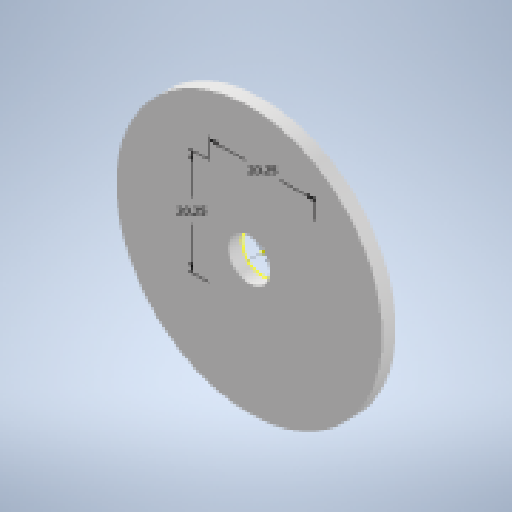
# Autodesk Inventor part: Base
Saved by Autodesk Inventor 2026 (Build 300175050, 175E)
## iProperties
Created: 2025-10-07
Part Number: Base
Material: Generic
Document SubType Name: Modeling
Designer: Cupri
Density: 1 g/cm^3
Appearance: Default
Author: Cupri
Autodesk Inventor part; units mm, degrees
ref_plane "YZ Plane" through (0, 0, 0) normal (1, 0, 0) x (0, 1, 0)
ref_plane "XZ Plane" through (0, 0, 0) normal (0, 1, 0) x (-1, 0, 0)
sketch "Sketch1" plane through (0, 0, 0) normal (0, 0, 1) x (1, 0, 0)
  line L0 (-25.4, 25.4) -> (25.4, 25.4)
  line L1 (25.4, 25.4) -> (25.4, -25.4)
  line L2 (25.4, -25.4) -> (-25.4, -25.4)
  line L3 (-25.4, -25.4) -> (-25.4, 25.4)
  line L4 (-25.4, 25.4) -> (25.4, -25.4) construction
  line L5 (25.4, 25.4) -> (-25.4, -25.4) construction
  circle A0 centre (0, 0) radius 25.4
  dimension "d0" = 50.8
  dimension "d1" = 50.8
  constraints: 12 end point, 2 midpoint, 2 parallel, 1 centre point, 1 coincident, 1 horizontal, 1 perpendicular
  measures "d0" distance of L1.end L2.end
  measures "d1" distance of L0.end L1.end
extrude "Extrusion1" add sketch "Sketch1" along normal blind 2.54 contours A0
sketch "Sketch2" plane through (0, 0, 2.54) normal (0, 0, 1) x (1, 0, 0)
  circle A0 centre (0, 0) radius 3.975 projected
extrude "Extrusion2" cut sketch "Sketch2" against normal blind 2.54
sketch "Sketch3" plane through (0, 0, 0) normal (0, 0, -1) x (-1, 0, 0)
  line L0 (-10, 10) -> (-10, -10) projected
  line L1 (10, 9.9) -> (10, -9.9) projected
  line L2 (7, -10) -> (-7, -10) projected
  line L3 (-7, 10) -> (7, 10) projected
  line L4 (-10.125, -10.125) -> (10.125, -10.125)
  line L5 (10.125, -10.125) -> (10.125, 10.125)
  line L6 (10.125, 10.125) -> (-10.125, 10.125)
  line L7 (-10.125, 10.125) -> (-10.125, -10.125)
  line L8 (-10.125, -10.125) -> (10.125, 10.125) construction
  line L9 (10.125, -10.125) -> (-10.125, 10.125) construction
  circle A0 centre (0, 0) radius 3.975 projected
  circle A1 centre (0, 0) radius 3.975 projected
  circle A2 centre (0, 0) radius 25.4 projected
  dimension "d6" = 20.25
  dimension "d7" = 20.25
  constraints: 12 end point, 2 midpoint, 2 parallel, 1 horizontal, 1 perpendicular
  measures "d6" distance of L6.end L5.end
  measures "d7" distance of L5.end L4.end
ref_plane "Work Plane1" through (7, -9.9, -1.8716) normal (0, 0, -1) x (0, 1, 0)
extrude "Extrusion3" add sketch "Sketch3" along normal up to surface (1.8716 mm away) contours A2
body "Solid1"
